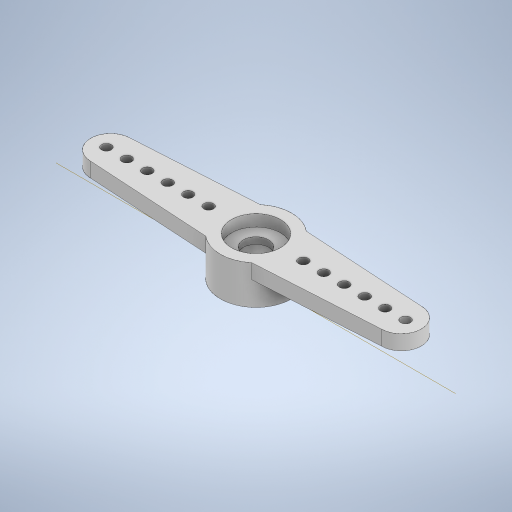
# Autodesk Inventor part: Servo Horn
Saved by Autodesk Inventor 2023 (Build 270158000, 158)
## iProperties
Created: 2023-03-10
Part Number: Servo Horn
Material: Generic
Document SubType Name: Modeling
Designer: 1ROWESTE
Density: 1 g/cm^3
Appearance: Default
Author: 1ROWESTE
Autodesk Inventor part; units mm, degrees
ref_plane "YZ Plane" through (0, 0, 0) normal (1, 0, 0) x (0, 1, 0)
ref_plane "XZ Plane" through (0, 0, 0) normal (0, 1, 0) x (-1, 0, 0)
ref_plane "XY Plane" through (0, 0, 0) normal (0, 0, 1) x (1, 0, 0)
sketch "Sketch1" plane through (0, 0, 0) normal (0, 1, 0) x (-1, 0, 0)
  circle A0 centre (0, 0) radius 2.375
  circle A1 centre (0, 0) radius 3.45
  dimension "d0" = 4.75
  dimension "d1" = 6.9
  constraints: 2 centre point, 2 coincident
  measures "d0" diameter of A0
  measures "d1" diameter of A1
extrude "Extrusion1" add sketch "Sketch1" along normal blind 3.75
ref_plane "2mm deep in well" through (0, 2, 0) normal (0, -1, 0) x (1, 0, 0)
sketch "Sketch2" plane through (0, 2, 0) normal (0, -1, 0) x (1, 0, 0)
  point P0 (0, 0)
sketch "Sketch3" plane through (0, 2, 0) normal (0, -1, 0) x (1, 0, 0)
  circle A0 centre (0, 0) radius 3.45 projected
  circle A1 centre (0, 0) radius 2.375 projected
  circle A2 centre (0, 0) radius 1.215
  dimension "d5" = 2.43
  constraints: 1 centre point, 1 coincident
  measures "d5" diameter of A2
extrude "Extrusion2" add sketch "Sketch3" against normal blind 0.63 contours A1
sketch "Sketch4" plane through (0, 3.75, 0) normal (0, 1, 0) x (1, 0, 0)
  line L0 (-16, 0) -> (16, 0)
  circle A0 centre (14.075, 0) radius 1.925
  circle A1 centre (0, 0) radius 3.45 projected
  circle A2 centre (0, 0) radius 2.375 projected
  line L1 (2.221, 2.64) -> (2.221, -2.64)
  line L2 (2.221, 2.64) -> (14.075, 1.925)
  line L3 (2.221, -2.64) -> (14.075, -1.925)
  dimension "d8" = 32
  dimension "d9" = 0
  dimension "d10" = 0
  dimension "d11" = 3.85
  dimension "d12" = 1.925
  dimension "d13" = 0
  dimension "d14" = 5.28
  constraints: 8 end point, 4 point on circle, 1 centre point, 1 horizontal, 1 midpoint, 1 perpendicular
  measures "d8" distance of L0.start L0.end
  measures "d9" distance of point (0, 0) point (0, 0)
  measures "d10" distance of point (0, 0) point (0, 0)
  measures "d11" diameter of A0
  measures "d12" distance of A0.centre L0.end
  measures "d13" distance from line of L0 A0.centre
  measures "d14" distance of L1.start L1.end
extrude "Extrusion3" add sketch "Sketch4" against normal blind 1.43 contours A1 L2 A0 L0 | L0 A0 L3 A1 | A0 L0 | L0 A0
sketch "Sketch5" plane through (0, 3.75, 0) normal (0, 1, 0) x (1, 0, 0)
  circle A0 centre (14.485, 0) radius 0.465
  arc A1 (2.221, 2.64) -> (2.221, -2.64) centre (0, 0) ccw projected
  line L0 (2.221, -2.64) -> (14.075, -1.925) projected
  arc A2 (14.075, -1.925) -> (14.075, 1.925) centre (14.075, 0) ccw projected
  line L1 (14.075, 1.925) -> (2.221, 2.64) projected
  circle A3 centre (0, 0) radius 2.375 projected
  point P0 (16, 0)
  dimension "d17" = 0.93
  dimension "d18" = 0
  dimension "d19" = 1.515
  constraints: 1 centre point, 1 point on circle
  measures "d17" diameter of A0
  measures "d18" vertical distance of A0.centre A2.centre
  measures "d19" distance of point (16, 0) A0.centre
extrude "Extrusion4" cut sketch "Sketch5" against normal up to surface (1.43 mm away) contours A0
pattern_linear "Rectangular Pattern1" count 6 spacing 1.98 along (-1, 0, 0) of "Extrusion4"
mirror "Mirror1" about plane through (0, 0, 0) normal (1, 0, 0) of "Extrusion3", "Extrusion4", "Rectangular Pattern1"
body "Solid1"
